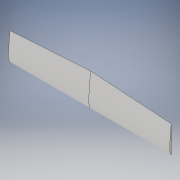
# Autodesk Inventor part: hTail_wing
Saved by Autodesk Inventor 2019 (Build 230136000, 136)
## iProperties
Created: 2019-04-06
Part Number: hTail_wing
Material: Generic
Document SubType Name: Modeling
Designer: albaa
Density: 0.03 g/cm^3
Appearance: Default
Author: albaa
Autodesk Inventor part; units mm, degrees
ref_plane "XZ Plane" through (0, 0, 0) normal (0, 1, 0) x (-1, 0, 0)
ref_plane "XY Plane" through (0, 0, 0) normal (0, 0, 1) x (1, 0, 0)
sketch "Sketch1" plane through (0, 0, 0) normal (1, 0, 0) x (0, 1, 0)
  spline S0 degree 5 poles (119.9226, 0.0645) (119.2502, 0.3016) (115.2909, 0.7762) (103.9493, 1.3369) (100.5816, 2.1691) (87.9343, 3.0641) (79.6308, 3.8887) (69.775, 4.6512) (60.9603, 5.3238) (52.3944, 5.8819) (44.4516, 6.3161) (37.05, 6.6056) (30.27, 6.7531) (24.1186, 6.7311) (18.6302, 6.6046) (13.8137, 5.9896) (9.7367, 5.2219) (6.3356, 4.2097) (3.7118, 3.2803) (1.6451, 2.1413) (0.3339, 1.2494) (-0.4685, -0.1076) (0.8297, -1.0394) (2.4385, -1.3568) (4.9268, -1.6981) (7.9154, -1.7449) (11.7917, -1.8163) (16.3299, -1.7732) (21.653, -1.7633) (27.619, -1.9273) (34.2298, -1.9754) (41.3809, -1.9166) (49.0549, -1.7774) (57.0835, -1.5625) (65.6444, -1.3277) (74.0565, -1.0198) (83.7807, -0.8527) (90.7752, -0.3942) (102.7184, -0.6765) (104.0081, 0.266) (116.259, -0.4711) (120.0255, -0.281) (120.2853, -0.0634) (119.9226, 0.0645) knots 0 0 0 0 0 0 0.041807 0.069402 0.10363 0.137323 0.170361 0.202622 0.233985 0.264329 0.293536 0.321494 0.348094 0.373231 0.396789 0.418625 0.438554 0.456334 0.471767 0.485224 0.497686 0.510232 0.523947 0.539825 0.558267 0.579063 0.60192 0.626577 0.652798 0.680373 0.709112 0.738839 0.769392 0.800622 0.832393 0.864574 0.897044 0.92968 0.956823 0.977448 1 1 1 1 1 1
  point P0 (0, 0)
  point P1 (0, 0)
  point P2 (0.248, 0.877)
  point P3 (1.3068, 1.8601)
  point P4 (3.1568, 2.912)
  point P5 (5.7771, 3.9757)
  point P6 (9.1463, 4.9766)
  point P7 (13.2433, 5.8267)
  point P8 (18.0482, 6.4288)
  point P9 (23.541, 6.6884)
  point P10 (29.7014, 6.7176)
  point P11 (36.5062, 6.5905)
  point P12 (43.9278, 6.3107)
  point P13 (51.932, 5.8874)
  point P14 (60.4766, 5.3343)
  point P15 (69.512, 4.6668)
  point P16 (78.9812, 3.9005)
  point P17 (88.8221, 3.0485)
  point P18 (98.9697, 2.1212)
  point P19 (0, 0)
  point P20 (0.5717, -0.7145)
  point P21 (1.9665, -1.2277)
  point P22 (4.1871, -1.5556)
  point P23 (7.2267, -1.7272)
  point P24 (11.0681, -1.785)
  point P25 (15.683, -1.7846)
  point P26 (21.0319, -1.7945)
  point P27 (27.0653, -1.8893)
  point P28 (33.7249, -1.9486)
  point P29 (40.9462, -1.9035)
  point P30 (48.6611, -1.7695)
  point P31 (56.8005, -1.5677)
  point P32 (65.296, -1.3218)
  point P33 (74.0811, -1.0567)
  point P34 (83.0909, -0.7948)
  point P35 (92.2614, -0.5546)
  point P36 (101.5276, -0.3493)
  point P37 (110.8229, -0.1855)
  point P38 (120.0774, -0.0645)
  constraints: 39 other
ref_plane "Work Plane1" through (300, 0, 0) normal (1, 0, 0) x (0, 1, 0)
sketch "Sketch2" plane through (300, 0, 0) normal (1, 0, 0) x (0, 1, 0)
  spline S0 degree 5 poles (99.9355, 0.0538) (99.3752, 0.2513) (96.0758, 0.6469) (86.6244, 1.1141) (83.818, 1.8076) (73.2786, 2.5534) (66.359, 3.2406) (58.1458, 3.876) (50.8002, 4.4365) (43.662, 4.9016) (37.043, 5.2634) (30.875, 5.5046) (25.225, 5.6276) (20.0988, 5.6092) (15.5252, 5.5038) (11.5114, 4.9913) (8.1139, 4.3515) (5.2797, 3.5081) (3.0932, 2.7336) (1.371, 1.7844) (0.2783, 1.0411) (-0.3904, -0.0897) (0.6915, -0.8662) (2.0321, -1.1307) (4.1057, -1.4151) (6.5961, -1.4541) (9.8264, -1.5136) (13.6083, -1.4777) (18.0442, -1.4694) (23.0159, -1.606) (28.5248, -1.6461) (34.4841, -1.5972) (40.8791, -1.4812) (47.5696, -1.3021) (54.7037, -1.1064) (61.7138, -0.8499) (69.8172, -0.7105) (75.646, -0.3285) (85.5987, -0.5638) (86.6734, 0.2216) (96.8825, -0.3926) (100.0213, -0.2342) (100.2377, -0.0528) (99.9355, 0.0538) knots 0 0 0 0 0 0 0.041807 0.069402 0.10363 0.137323 0.170361 0.202622 0.233985 0.264329 0.293536 0.321494 0.348094 0.373231 0.396789 0.418625 0.438554 0.456334 0.471767 0.485224 0.497686 0.510232 0.523947 0.539825 0.558267 0.579063 0.60192 0.626577 0.652798 0.680373 0.709112 0.738839 0.769392 0.800622 0.832393 0.864574 0.897044 0.92968 0.956823 0.977448 1 1 1 1 1 1
  point P0 (0, 0)
  point P1 (0, 0)
  point P2 (0.2067, 0.7308)
  point P3 (1.089, 1.5501)
  point P4 (2.6307, 2.4267)
  point P5 (4.8143, 3.3131)
  point P6 (7.6219, 4.1472)
  point P7 (11.0361, 4.8555)
  point P8 (15.0401, 5.3573)
  point P9 (19.6175, 5.5737)
  point P10 (24.7512, 5.598)
  point P11 (30.4219, 5.4921)
  point P12 (36.6065, 5.2589)
  point P13 (43.2766, 4.9062)
  point P14 (50.3972, 4.4452)
  point P15 (57.9267, 3.889)
  point P16 (65.8177, 3.2504)
  point P17 (74.0184, 2.5404)
  point P18 (82.4747, 1.7677)
  point P19 (0, 0)
  point P20 (0.4764, -0.5954)
  point P21 (1.6387, -1.0231)
  point P22 (3.4892, -1.2963)
  point P23 (6.0223, -1.4394)
  point P24 (9.2234, -1.4875)
  point P25 (13.0691, -1.4872)
  point P26 (17.5266, -1.4954)
  point P27 (22.5544, -1.5744)
  point P28 (28.1041, -1.6238)
  point P29 (34.1218, -1.5862)
  point P30 (40.5509, -1.4746)
  point P31 (47.3337, -1.3064)
  point P32 (54.4133, -1.1015)
  point P33 (61.7343, -0.8806)
  point P34 (69.2425, -0.6623)
  point P35 (76.8845, -0.4622)
  point P36 (84.6063, -0.291)
  point P37 (92.3524, -0.1546)
  point P38 (100.0645, -0.0538)
  constraints: 39 other
loft "Loft1" add profiles "Sketch1", "Sketch2"
mirror "Mirror1" about plane through (0, 59.3325, 1.3613) normal (-1, 0, 0) of "Loft1"
body "Solid1"
